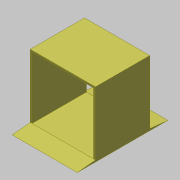
# Autodesk Inventor part: Tunnel
Saved by Autodesk Inventor 2015 (Build 190159000, 159)
## iProperties
Created: 2015-03-07
Part Number: Tunnel
Material: Generic
Document SubType Name: Modeling
Designer: Vukica
Density: 1 g/cm^3
Appearance: Plywood - Weathered
Author: Vukica
Autodesk Inventor part; units mm, degrees
ref_plane "YZ Plane" through (0, 0, 0) normal (1, 0, 0) x (0, 1, 0)
ref_plane "XZ Plane" through (0, 0, 0) normal (0, 1, 0) x (-1, 0, 0)
ref_plane "XY Plane" through (0, 0, 0) normal (0, 0, 1) x (1, 0, 0)
sketch "Sketch1" plane through (0, 0, 0) normal (0, 0, 1) x (1, 0, 0)
  line L0 (0, 0) -> (457.2, 0)
  line L1 (457.2, 0) -> (457.2, 457.2)
  line L2 (457.2, 457.2) -> (0, 457.2)
  line L3 (0, 457.2) -> (0, 0)
  dimension "d0" = 457.2
  dimension "d1" = 457.2
  constraints: 8 end point, 2 parallel, 1 horizontal, 1 perpendicular
  measures "d0" distance of L0.start L0.end
  measures "d1" distance of L2.end L0.start
extrude "Extrusion1" add sketch "Sketch1" along normal blind 381
shell "Shell1" thickness 12.7 removed faces 2 at (304.8, 152.4, 381) at (304.8, 152.4, 0)
sketch "Sketch2" plane through (457.2, 0, 0) normal (1, 0, 0) x (0, 0, -1)
  line L0 (0, 12.7) -> (-381, 12.7) projected
  line L1 (-381, 0) -> (-381, 457.2) projected
  line L2 (0, 0) -> (0, 457.2) projected
  line L3 (0, 0) -> (-381, 0) projected
  line L4 (-381, 12.7) -> (-508, 0)
  line L5 (-508, 0) -> (-381, 0)
  line L6 (-381, 12.7) -> (-381, 0)
  line L7 (0, 12.7) -> (0, 0)
  line L8 (127, 0) -> (0, 0)
  line L9 (0, 12.7) -> (127, 0)
  dimension "d9" = 127
  dimension "d10" = 127
  constraints: 12 end point, 2 perpendicular, 1 collinear, 1 horizontal
  measures "d9" distance of L4.end L1.start
  measures "d10" distance of L8.start L2.start
extrude "Extrusion2" add sketch "Sketch2" against normal up to surface (457.2 mm away) contours L9 L8 L2 | L1 L5 L4
equation "\"d1\" = d0"
body "Solid1"
